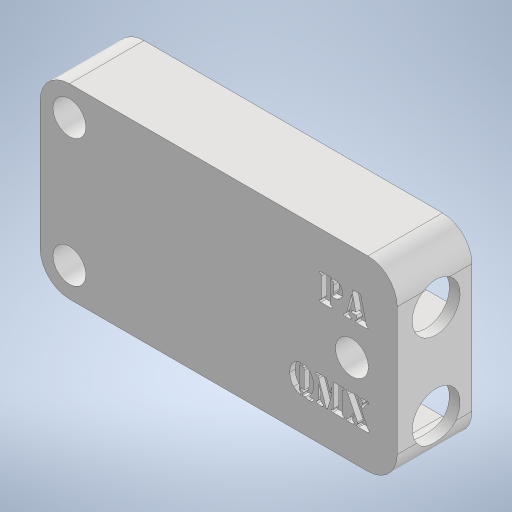
# Autodesk Inventor part: Case_Cap
Saved by Autodesk Inventor 2023 (Build 270158000, 158)
## iProperties
Created: 2024-10-24
Part Number: Case_Cap
Material: Generic
Document SubType Name: Modeling
Designer: lwerne
Density: 1 g/cm^3
Appearance: Default
Author: lwerne
Autodesk Inventor part; units mm, degrees
ref_plane "YZ Plane" through (0, 0, 0) normal (1, 0, 0) x (0, 1, 0)
ref_plane "XZ Plane" through (0, 0, 0) normal (0, 1, 0) x (-1, 0, 0)
ref_plane "XY Plane" through (0, 0, 0) normal (0, 0, 1) x (1, 0, 0)
sketch "Sketch1" plane through (0, 0, 0) normal (0, 0, 1) x (1, 0, 0)
  arc A0 (31.5, 12) -> (28, 15.5) centre (28, 12) ccw projected
  line L0 (31.5, 12) -> (31.5, -12) projected
  arc A1 (28, -15.5) -> (31.5, -12) centre (28, -12) ccw projected
  line L1 (28, -15.5) -> (-28, -15.5) projected
  arc A2 (-31.5, -12) -> (-28, -15.5) centre (-28, -12) ccw projected
  line L2 (-31.5, -12) -> (-31.5, 12) projected
  arc A3 (-28, 15.5) -> (-31.5, 12) centre (-28, 12) ccw projected
  line L3 (-28, 15.5) -> (28, 15.5) projected
  arc A4 (28, -17.5) -> (33.5, -12) centre (28, -12) ccw projected
  line L4 (33.5, 12) -> (33.5, -12) projected
  arc A5 (33.5, 12) -> (28, 17.5) centre (28, 12) ccw projected
  line L5 (-28, 17.5) -> (28, 17.5) projected
  arc A6 (-28, 17.5) -> (-33.5, 12) centre (-28, 12) ccw projected
  line L6 (-33.5, -12) -> (-33.5, 12) projected
  arc A7 (-33.5, -12) -> (-28, -17.5) centre (-28, -12) ccw projected
  line L7 (28, -17.5) -> (-28, -17.5) projected
  point P0 (0, 0)
extrude "Extrusion1" add sketch "Sketch1" along normal blind 12
ref_plane "Work Plane1" through (0, 0, 5.9) normal (0, 0, 1) x (1, 0, 0)
sketch "Sketch2" plane through (0, 0, 5.9) normal (0, 0, 1) x (1, 0, 0)
  circle A0 centre (-28, 12) radius 1.6 projected
  circle A1 centre (-28, -12) radius 1.6 projected
  circle A2 centre (25, -0.5) radius 1.6 projected
  line L0 (-28, 15.5) -> (28, 15.5) projected
  circle A3 centre (-28, 12) radius 3.5
  circle A4 centre (-28, -12) radius 3.5
  circle A5 centre (25, -0.5) radius 4
  line L1 (25, 3.5) -> (31.5, 3.5)
  line L2 (31.5, 12) -> (31.5, -12) projected
  line L3 (25, -4.5) -> (31.5, -4.5)
  line L4 (-28, -17.5) -> (28, -17.5) projected
  arc A6 (28, -17.5) -> (33.5, -12) centre (28, -12) ccw projected
  line L5 (33.5, -12) -> (33.5, 12) projected
  arc A7 (33.5, 12) -> (28, 17.5) centre (28, 12) ccw projected
  line L6 (28, 17.5) -> (-28, 17.5) projected
  arc A8 (-28, 17.5) -> (-33.5, 12) centre (-28, 12) ccw projected
  line L7 (-33.5, 12) -> (-33.5, -12) projected
  arc A9 (-33.5, -12) -> (-28, -17.5) centre (-28, -12) ccw projected
  line L8 (28, -15.5) -> (-28, -15.5) projected
  arc A10 (-31.5, -12) -> (-28, -15.5) centre (-28, -12) ccw projected
  line L9 (-31.5, -12) -> (-31.5, 12) projected
  arc A11 (-28, 15.5) -> (-31.5, 12) centre (-28, 12) ccw projected
  line L10 (-28, 15.5) -> (28, 15.5) projected
  arc A12 (31.5, 12) -> (28, 15.5) centre (28, 12) ccw projected
  line L11 (31.5, 12) -> (31.5, -12) projected
  arc A13 (28, -15.5) -> (31.5, -12) centre (28, -12) ccw projected
  circle A14 centre (-28, 12) radius 5.5
  circle A15 centre (-28, -12) radius 5.5
  point P0 (0, 0)
  point P1 (-23.7574, -15.5)
  point P2 (-31.5, -7.7574)
  point P3 (-31.5, 7.7574)
  point P4 (-23.7574, 15.5)
  point P5 (-31.5, 12)
  dimension "d2" = 8
  constraints: 4 centre point, 4 end point, 3 coincident, 2 point on circle, 2 point on line, 1 horizontal, 1 parallel, 3 other
  measures "d2" diameter of A5
ref_plane "Work Plane2" through (-31, -15, 0) normal (0, 0, 1) x (1, 0, 0)
extrude "Extrusion2" add sketch "Sketch2" against normal up to surface (5.9 mm away) contours L0 A14 L9 A3 | A3 | A15 L8 A4 L9 | L2 L3 A5 L1 | A4 | A5
sketch "Sketch3" plane through (0, 0, 5.9) normal (0, 0, 1) x (1, 0, 0)
  circle A0 centre (-28, 12) radius 1.6 projected
  circle A1 centre (-28, -12) radius 1.6 projected
  circle A2 centre (25, -0.5) radius 1.6 projected
  circle A3 centre (-28, 12) radius 3.1
  circle A4 centre (-28, -12) radius 1.6 projected
  circle A5 centre (-28, -12) radius 3.1
  circle A6 centre (25, -0.5) radius 1.6 projected
  circle A7 centre (25, -0.5) radius 3.1
  line L0 (31.5, 3.5) -> (31.5, -4.5) projected
  line L1 (31.5, 3.5) -> (25, 3.5) projected
  arc A8 (25, 3.5) -> (25, -4.5) centre (25, -0.5) ccw projected
  line L2 (25, -4.5) -> (31.5, -4.5) projected
  circle A9 centre (25, -0.5) radius 1.6 projected
  arc A10 (-31.5, -12) -> (-28, -15.5) centre (-28, -12) ccw projected
  circle A11 centre (-28, -12) radius 1.6 projected
  arc A12 (-28, 15.5) -> (-31.5, 12) centre (-28, 12) ccw projected
  circle A13 centre (-28, 12) radius 1.6 projected
  line L3 (-31.5, 7.7574) -> (-31.5, 12) projected
  arc A14 (-31.5, 7.7574) -> (-23.7574, 15.5) centre (-28, 12) ccw projected
  line L4 (-28, 15.5) -> (-23.7574, 15.5) projected
  line L5 (-23.7574, -15.5) -> (-28, -15.5) projected
  arc A15 (-23.7574, -15.5) -> (-31.5, -7.7574) centre (-28, -12) ccw projected
  line L6 (-31.5, -12) -> (-31.5, -7.7574) projected
  point P0 (0, 0)
  dimension "d5" = 6.2
  dimension "d6" = 6.2
  dimension "d7" = 6.2
  constraints: 3 centre point, 3 coincident
  measures "d5" diameter of A3
  measures "d6" diameter of A5
  measures "d7" diameter of A7
extrude "Extrusion3" add sketch "Sketch3" along normal up to surface (6.1 mm away) contours L0 L2 A8 L1 | L6 A15 L5 A10 | L4 A14 L3 A12
fillet "Fillet1" radius 2 4 edges at (-23.7574, -15.5, 6) (-31.5, -7.7574, 6) (-31.5, 7.7574, 6) (-23.7574, 15.5, 6)
sketch "Sketch4" plane through (0, 0, 12) normal (0, 0, 1) x (1, 0, 0)
  circle A0 centre (25, -0.5) radius 3.1 projected
  circle A1 centre (-28, 12) radius 3.1 projected
  circle A2 centre (-28, -12) radius 3.1 projected
  line L0 (-28, -17.5) -> (28, -17.5) projected
  arc A3 (28, -17.5) -> (33.5, -12) centre (28, -12) ccw projected
  line L1 (33.5, -12) -> (33.5, 12) projected
  arc A4 (33.5, 12) -> (28, 17.5) centre (28, 12) ccw projected
  line L2 (28, 17.5) -> (-28, 17.5) projected
  arc A5 (-28, 17.5) -> (-33.5, 12) centre (-28, 12) ccw projected
  line L3 (-33.5, 12) -> (-33.5, -12) projected
  arc A6 (-33.5, -12) -> (-28, -17.5) centre (-28, -12) ccw projected
  line L4 (-31.5, -4.6515) -> (-31.5, 4.6515) projected
  arc A7 (-29.1, 6.6111) -> (-31.5, 4.6515) centre (-29.5, 4.6515) ccw projected
  arc A8 (-29.1, 6.6111) -> (-22.6111, 13.1) centre (-28, 12) ccw projected
  arc A9 (-20.6515, 15.5) -> (-22.6111, 13.1) centre (-20.6515, 13.5) ccw projected
  line L5 (-20.6515, 15.5) -> (28, 15.5) construction
  arc A10 (31.5, 12) -> (28, 15.5) centre (28, 12) ccw projected
  line L6 (31.5, 12) -> (31.5, 3.5) projected
  line L7 (25, 3.5) -> (31.5, 3.5) projected
  arc A11 (25, 3.5) -> (25, -4.5) centre (25, -0.5) ccw projected
  line L8 (31.5, -4.5) -> (25, -4.5) projected
  line L9 (31.5, -4.5) -> (31.5, -12) projected
  arc A12 (28, -15.5) -> (31.5, -12) centre (28, -12) ccw projected
  line L10 (28, -15.5) -> (-20.6515, -15.5) projected
  arc A13 (-22.6111, -13.1) -> (-20.6515, -15.5) centre (-20.6515, -13.5) ccw projected
  arc A14 (-22.6111, -13.1) -> (-29.1, -6.6111) centre (-28, -12) ccw projected
  arc A15 (-31.5, -4.6515) -> (-29.1, -6.6111) centre (-29.5, -4.6515) ccw projected
  point P0 (0, 0)
sketch "Sketch5" plane through (0, 0, 12) normal (0, 0, 1) x (1, 0, 0)
  point P0 (0, 0)
extrude "Extrusion4" add sketch "Sketch4" along normal blind 2
sketch "Sketch6" plane through (33.5, -12, 0) normal (1, 0, 0) x (0, 0, -1)
  circle A0 centre (-6.7, 2.595) radius 3.2 projected
  circle A1 centre (-6.7, 20.267) radius 3.2 projected
  circle A2 centre (-6.7, 2.595) radius 4.5
  circle A3 centre (-6.7, 20.267) radius 4.5
  point P0 (0, 12)
  dimension "d13" = 9
  dimension "d14" = 9
  constraints: 2 centre point, 2 coincident
  measures "d13" diameter of A2
  measures "d14" diameter of A3
extrude "Extrusion5" cut sketch "Sketch6" against normal blind 5.9375 contours A0 | A1 | A2 | A3
sketch "Sketch7" plane through (-33.5, -12, 0) normal (-1, 0, 0) x (0, 0, 1)
  arc A0 (1.2, 17.6122) -> (0.07, 16.4822) centre (1.2, 16.4822) ccw projected
  arc A1 (0.07, 10.0022) -> (1.2, 8.8722) centre (1.2, 10.0022) ccw projected
  arc A2 (1.9, 8.8722) -> (3.03, 10.0022) centre (1.9, 10.0022) ccw projected
  line L0 (0, 13.1) -> (5.9, 13.1) projected
  line L1 (0, 24) -> (0, 0) projected
  line L2 (0, 7.3485) -> (0, 16.6515) projected
  line L3 (0, 17.6122) -> (0, 8.8722)
  line L4 (0, 8.8722) -> (3.03, 8.8722)
  line L5 (3.03, 8.8722) -> (3.03, 17.6122)
  line L6 (3.03, 17.6122) -> (0, 17.6122)
  line L7 (-2.485, 20.7422) -> (5.515, 20.7422)
  line L8 (5.515, 20.7422) -> (5.515, 5.7422)
  line L9 (5.515, 5.7422) -> (-2.485, 5.7422)
  line L10 (-2.485, 5.7422) -> (-2.485, 20.7422)
  line L11 (-2.485, 20.7422) -> (5.515, 5.7422) construction
  line L12 (5.515, 20.7422) -> (-2.485, 5.7422) construction
  point P0 (1.515, 13.2422)
  point P1 (0, 5.7422)
  point P2 (0, 20.7422)
  dimension "d17" = 8
  dimension "d18" = 15
  constraints: 20 end point, 4 parallel, 2 midpoint, 2 perpendicular, 2 point on line, 1 horizontal
  measures "d17" distance of L8.end L9.end
  measures "d18" distance of L7.end L8.end
extrude "Extrusion6" cut sketch "Sketch7" against normal blind 11.525 contours L4 L1 L0 L5 A2 | L4 L5 L0 L8 L9 L1 | A2 L5 L4 | L5 L6 L1 L7 L8 L0 | L0 L1 L6 L5
fillet "Fillet2" radius 2 2 edges at (-28.5343, 8.7422, 5.515) (-32.0958, -6.2578, 5.515)
sketch "Sketch8" plane through (0, 0, 14) normal (0, 0, 1) x (1, 0, 0)
  line L0 (13.173, -6.1079) -> (28.4117, -6.1079) construction
  line L1 (28.4117, -6.1079) -> (28.4117, -11.4638) construction
  line L2 (28.4117, -11.4638) -> (13.173, -11.4638) construction
  line L3 (13.173, -11.4638) -> (13.173, -6.1079) construction
  line L4 (18.6124, 10.5749) -> (28.0308, 10.5749) construction
  line L5 (28.0308, 10.5749) -> (28.0308, 5.5749) construction
  line L6 (28.0308, 5.5749) -> (18.6124, 5.5749) construction
  line L7 (18.6124, 5.5749) -> (18.6124, 10.5749) construction
  line L8 (20.9127, 10.5749) -> (20.9127, 6.2693)
  spline S0 degree 2 poles (20.9127, 6.2693) (20.9127, 6.1261) (20.9692, 6.0653) knots 0 0 0 1 1 1
  spline S1 degree 2 poles (20.9692, 6.0653) (20.9952, 6.0306) (21.0473, 6.0089) (21.1905, 5.9742) knots 0 0 0 1 2 2 2
  spline S2 degree 2 poles (21.1905, 5.9742) (21.3685, 5.9351) (21.3685, 5.7745) knots 0 0 0 1 1 1
  spline S3 degree 2 poles (21.3685, 5.7745) (21.3685, 5.679) (21.273, 5.6183) knots 0 0 0 1 1 1
  spline S4 degree 2 poles (21.273, 5.6183) (21.2035, 5.5749) (21.0429, 5.5749) knots 0 0 0 1 1 1
  line L9 (21.0429, 5.5749) -> (20.9171, 5.5749)
  line L10 (20.9171, 5.5749) -> (19.2808, 5.5749)
  line L11 (19.2808, 5.5749) -> (19.1853, 5.5749)
  spline S5 degree 2 poles (19.1853, 5.5749) (19.0551, 5.5749) (18.9119, 5.6747) (18.9119, 5.7658) knots 0 0 0 1 2 2 2
  spline S6 degree 2 poles (18.9119, 5.7658) (18.9119, 5.9134) (19.0594, 5.9612) knots 0 0 0 1 1 1
  spline S7 degree 2 poles (19.0594, 5.9612) (19.181, 6.0046) (19.22, 6.0219) (19.2417, 6.0566) knots 0 0 0 1 2 2 2
  spline S8 degree 2 poles (19.2417, 6.0566) (19.2851, 6.1131) (19.2851, 6.2433) knots 0 0 0 1 1 1
  line L12 (19.2851, 6.2433) -> (19.2851, 9.9065)
  spline S9 degree 2 poles (19.2851, 9.9065) (19.2851, 10.0367) (19.2417, 10.0931) knots 0 0 0 1 1 1
  spline S10 degree 2 poles (19.2417, 10.0931) (19.22, 10.1278) (19.181, 10.1452) (19.0594, 10.1842) knots 0 0 0 1 2 2 2
  spline S11 degree 2 poles (19.0594, 10.1842) (18.9119, 10.232) (18.9119, 10.3839) knots 0 0 0 1 1 1
  spline S12 degree 2 poles (18.9119, 10.3839) (18.9119, 10.475) (19.0551, 10.5749) (19.1853, 10.5749) knots 0 0 0 1 2 2 2
  line L13 (19.1853, 10.5749) -> (19.2808, 10.5749)
  line L14 (19.2808, 10.5749) -> (20.9127, 10.5749)
  line L15 (21.2252, 7.4889) -> (21.2252, 7.8796)
  spline S13 degree 2 poles (21.2252, 7.8796) (21.3815, 7.9186) (21.5073, 7.9967) (21.5551, 8.0836) knots 0 0 0 1 2 2 2
  spline S14 degree 2 poles (21.5551, 8.0836) (21.6332, 8.2268) (21.6332, 8.4655) knots 0 0 0 1 1 1
  line L16 (21.6332, 8.4655) -> (21.6332, 9.6417)
  spline S15 degree 2 poles (21.6332, 9.6417) (21.6332, 9.8153) (21.5811, 9.9803) (21.503, 10.0497) knots 0 0 0 1 2 2 2
  spline S16 degree 2 poles (21.503, 10.0497) (21.3988, 10.1539) (21.2209, 10.1799) knots 0 0 0 1 1 1
  line L17 (21.2209, 10.1799) -> (21.2209, 10.5749)
  spline S17 degree 2 poles (21.2209, 10.5749) (21.9761, 10.5749) (22.332, 10.4316) knots 0 0 0 1 1 1
  spline S18 degree 2 poles (22.332, 10.4316) (22.7487, 10.2667) (22.9874, 9.9282) knots 0 0 0 1 1 1
  spline S19 degree 2 poles (22.9874, 9.9282) (23.2348, 9.5766) (23.2348, 9.0731) knots 0 0 0 1 1 1
  spline S20 degree 2 poles (23.2348, 9.0731) (23.2348, 8.5089) (22.9874, 8.1487) knots 0 0 0 1 1 1
  spline S21 degree 2 poles (22.9874, 8.1487) (22.7356, 7.7928) (22.2886, 7.6235) knots 0 0 0 1 1 1
  spline S22 degree 2 poles (22.2886, 7.6235) (21.9197, 7.4889) (21.2252, 7.4889) knots 0 0 0 1 1 1
  line L18 (25.1575, 10.5749) -> (26.6332, 10.5749)
  line L19 (26.6332, 10.5749) -> (27.6488, 6.2693)
  spline S23 degree 2 poles (27.6488, 6.2693) (27.6792, 6.1565) (27.7139, 6.0697) knots 0 0 0 1 1 1
  spline S24 degree 2 poles (27.7139, 6.0697) (27.7487, 6.0002) (27.8615, 5.9568) knots 0 0 0 1 1 1
  spline S25 degree 2 poles (27.8615, 5.9568) (27.957, 5.9134) (28.0308, 5.8353) (28.0308, 5.7658) knots 0 0 0 1 2 2 2
  spline S26 degree 2 poles (28.0308, 5.7658) (28.0308, 5.5749) (27.7443, 5.5749) knots 0 0 0 1 1 1
  line L20 (27.7443, 5.5749) -> (25.9171, 5.5749)
  spline S27 degree 2 poles (25.9171, 5.5749) (25.8086, 5.5749) (25.674, 5.6834) (25.674, 5.7702) knots 0 0 0 1 2 2 2
  spline S28 degree 2 poles (25.674, 5.7702) (25.674, 5.844) (25.7348, 5.9178) (25.8346, 5.9698) knots 0 0 0 1 2 2 2
  spline S29 degree 2 poles (25.8346, 5.9698) (25.9084, 6.0089) (25.9692, 6.0957) (25.9692, 6.1608) knots 0 0 0 1 2 2 2
  spline S30 degree 2 poles (25.9692, 6.1608) (25.9692, 6.2259) (25.9561, 6.2737) knots 0 0 0 1 1 1
  line L21 (25.9561, 6.2737) -> (25.8389, 6.8032)
  line L22 (25.8389, 6.8032) -> (24.819, 6.8032)
  line L23 (24.819, 6.8032) -> (24.9188, 7.2372)
  line L24 (24.9188, 7.2372) -> (25.7391, 7.2372)
  line L25 (25.7391, 7.2372) -> (25.062, 10.2146)
  line L26 (25.062, 10.2146) -> (25.1575, 10.5749)
  line L27 (24.9014, 9.6417) -> (25.0881, 8.8865)
  line L28 (25.0881, 8.8865) -> (24.4414, 6.5211)
  spline S31 degree 2 poles (24.4414, 6.5211) (24.411, 6.4169) (24.411, 6.3301) knots 0 0 0 1 1 1
  spline S32 degree 2 poles (24.411, 6.3301) (24.411, 6.1) (24.628, 6.0002) knots 0 0 0 1 1 1
  line L29 (24.628, 6.0002) -> (24.7539, 5.9395)
  spline S33 degree 2 poles (24.7539, 5.9395) (24.8754, 5.8874) (24.8754, 5.7572) knots 0 0 0 1 1 1
  spline S34 degree 2 poles (24.8754, 5.7572) (24.8754, 5.5749) (24.6106, 5.5749) knots 0 0 0 1 1 1
  line L30 (24.6106, 5.5749) -> (23.6818, 5.5749)
  spline S35 degree 2 poles (23.6818, 5.5749) (23.5429, 5.5749) (23.3867, 5.6877) (23.3867, 5.7875) knots 0 0 0 1 2 2 2
  spline S36 degree 2 poles (23.3867, 5.7875) (23.3867, 5.8917) (23.5473, 5.9612) knots 0 0 0 1 1 1
  spline S37 degree 2 poles (23.5473, 5.9612) (23.6992, 6.0306) (23.8424, 6.1348) (23.9075, 6.2259) knots 0 0 0 1 2 2 2
  spline S38 degree 2 poles (23.9075, 6.2259) (24.0073, 6.3778) (24.0768, 6.6252) knots 0 0 0 1 1 1
  line L31 (24.0768, 6.6252) -> (24.9014, 9.6417)
  spline S39 degree 2 poles (16.9881, -10.7911) (17.1227, -10.9256) (17.344, -10.9256) knots 0 0 0 1 1 1
  spline S40 degree 2 poles (17.344, -10.9256) (17.4742, -10.9256) (17.5784, -10.8779) knots 0 0 0 1 1 1
  spline S41 degree 2 poles (17.5784, -10.8779) (17.6695, -10.8388) (17.7043, -10.8388) knots 0 0 0 1 1 1
  spline S42 degree 2 poles (17.7043, -10.8388) (17.7477, -10.8388) (17.8258, -10.9386) (17.8258, -10.9951) knots 0 0 0 1 2 2 2
  spline S43 degree 2 poles (17.8258, -10.9951) (17.8258, -11.1122) (17.6522, -11.2424) knots 0 0 0 1 1 1
  spline S44 degree 2 poles (17.6522, -11.2424) (17.3353, -11.4638) (17.0011, -11.4638) knots 0 0 0 1 1 1
  spline S45 degree 2 poles (17.0011, -11.4638) (16.5628, -11.4638) (16.3023, -11.1947) knots 0 0 0 1 1 1
  spline S46 degree 2 poles (16.3023, -11.1947) (16.055, -11.2815) (15.7208, -11.3119) knots 0 0 0 1 1 1
  line L32 (15.7208, -11.3119) -> (15.7208, -10.9039)
  spline S47 degree 2 poles (15.7208, -10.9039) (15.8032, -10.8865) (15.8813, -10.8431) (15.9291, -10.7997) knots 0 0 0 1 2 2 2
  line L33 (15.9291, -10.7997) -> (15.8987, -10.7694)
  spline S48 degree 2 poles (15.8987, -10.7694) (15.7989, -10.6478) (15.673, -10.5567) (15.5862, -10.5437) knots 0 0 0 1 2 2 2
  spline S49 degree 2 poles (15.5862, -10.5437) (15.4734, -10.5176) (15.4126, -10.4959) (15.3865, -10.4612) knots 0 0 0 1 2 2 2
  spline S50 degree 2 poles (15.3865, -10.4612) (15.3518, -10.4178) (15.3518, -10.357) knots 0 0 0 1 1 1
  spline S51 degree 2 poles (15.3518, -10.357) (15.3518, -10.2529) (15.5298, -10.1357) (15.6773, -10.1357) knots 0 0 0 1 2 2 2
  spline S52 degree 2 poles (15.6773, -10.1357) (15.7989, -10.1357) (15.9725, -10.1791) (16.068, -10.2355) knots 0 0 0 1 2 2 2
  line L34 (16.068, -10.2355) -> (16.068, -7.0194)
  spline S53 degree 2 poles (16.068, -7.0194) (16.068, -6.824) (16.0029, -6.7112) knots 0 0 0 1 1 1
  spline S54 degree 2 poles (16.0029, -6.7112) (15.9551, -6.6331) (15.8336, -6.5463) (15.7208, -6.5029) knots 0 0 0 1 2 2 2
  line L35 (15.7208, -6.5029) -> (15.7208, -6.1079)
  spline S55 degree 2 poles (15.7208, -6.1079) (16.1157, -6.1253) (16.7754, -6.4117) (17.0576, -6.6895) knots 0 0 0 1 2 2 2
  spline S56 degree 2 poles (17.0576, -6.6895) (17.8041, -7.4187) (17.8041, -8.7164) knots 0 0 0 1 1 1
  spline S57 degree 2 poles (17.8041, -8.7164) (17.8041, -10.0532) (16.9881, -10.7911) knots 0 0 0 1 1 1
  spline S58 degree 2 poles (15.4213, -6.5029) (15.2346, -6.5723) (15.0827, -6.798) (15.0827, -7.0194) knots 0 0 0 1 2 2 2
  line L36 (15.0827, -7.0194) -> (15.0827, -10.2919)
  spline S59 degree 2 poles (15.0827, -10.2919) (15.0827, -10.6131) (15.1695, -10.7477) knots 0 0 0 1 1 1
  spline S60 degree 2 poles (15.1695, -10.7477) (15.239, -10.8562) (15.4213, -10.9039) knots 0 0 0 1 1 1
  line L37 (15.4213, -10.9039) -> (15.4213, -11.3076)
  spline S61 degree 2 poles (15.4213, -11.3076) (14.6096, -11.2424) (14.0584, -10.6956) knots 0 0 0 1 1 1
  spline S62 degree 2 poles (14.0584, -10.6956) (13.3466, -9.9838) (13.3466, -8.7121) knots 0 0 0 1 1 1
  spline S63 degree 2 poles (13.3466, -8.7121) (13.3466, -8.074) (13.7242, -7.0454) (14.0931, -6.6895) knots 0 0 0 1 2 2 2
  spline S64 degree 2 poles (14.0931, -6.6895) (14.3753, -6.4117) (15.0263, -6.1253) (15.4213, -6.1079) knots 0 0 0 1 2 2 2
  line L38 (15.4213, -6.1079) -> (15.4213, -6.5029)
  line L39 (21.5454, -6.2077) -> (23.173, -6.2077)
  line L40 (23.173, -6.2077) -> (23.2728, -6.2077)
  spline S65 degree 2 poles (23.2728, -6.2077) (23.5463, -6.2077) (23.5463, -6.3987) knots 0 0 0 1 1 1
  spline S66 degree 2 poles (23.5463, -6.3987) (23.5463, -6.5506) (23.3987, -6.5984) knots 0 0 0 1 1 1
  spline S67 degree 2 poles (23.3987, -6.5984) (23.2772, -6.6374) (23.2381, -6.6548) (23.2164, -6.6895) knots 0 0 0 1 2 2 2
  spline S68 degree 2 poles (23.2164, -6.6895) (23.173, -6.7459) (23.173, -6.8761) knots 0 0 0 1 1 1
  line L41 (23.173, -6.8761) -> (23.173, -10.5393)
  spline S69 degree 2 poles (23.173, -10.5393) (23.173, -10.6695) (23.2164, -10.726) knots 0 0 0 1 1 1
  spline S70 degree 2 poles (23.2164, -10.726) (23.2381, -10.7607) (23.2772, -10.778) (23.3987, -10.8214) knots 0 0 0 1 2 2 2
  spline S71 degree 2 poles (23.3987, -10.8214) (23.5463, -10.8692) (23.5463, -11.0168) knots 0 0 0 1 1 1
  spline S72 degree 2 poles (23.5463, -11.0168) (23.5463, -11.2077) (23.2728, -11.2077) knots 0 0 0 1 1 1
  line L42 (23.2728, -11.2077) -> (23.173, -11.2077)
  line L43 (23.173, -11.2077) -> (21.5411, -11.2077)
  line L44 (21.5411, -11.2077) -> (21.4195, -11.2077)
  spline S73 degree 2 poles (21.4195, -11.2077) (21.2589, -11.2077) (21.094, -11.1079) (21.094, -11.0081) knots 0 0 0 1 2 2 2
  spline S74 degree 2 poles (21.094, -11.0081) (21.094, -10.8475) (21.272, -10.8084) knots 0 0 0 1 1 1
  spline S75 degree 2 poles (21.272, -10.8084) (21.4152, -10.7737) (21.4629, -10.752) (21.489, -10.7216) knots 0 0 0 1 2 2 2
  spline S76 degree 2 poles (21.489, -10.7216) (21.5454, -10.6565) (21.5454, -10.5133) knots 0 0 0 1 1 1
  line L45 (21.5454, -10.5133) -> (21.5454, -6.2077)
  line L46 (20.1999, -6.2077) -> (20.9247, -8.265)
  line L47 (20.9247, -8.265) -> (21.2416, -7.1539)
  line L48 (21.2416, -7.1539) -> (21.2416, -8.3692)
  line L49 (21.2416, -8.3692) -> (20.3952, -11.2077)
  line L50 (20.3952, -11.2077) -> (20.1999, -11.2077)
  line L51 (20.1999, -11.2077) -> (18.7806, -6.9933)
  spline S77 degree 2 poles (18.7806, -6.9933) (18.7069, -6.7806) (18.6287, -6.7069) knots 0 0 0 1 1 1
  spline S78 degree 2 poles (18.6287, -6.7069) (18.581, -6.6591) (18.4638, -6.6374) knots 0 0 0 1 1 1
  spline S79 degree 2 poles (18.4638, -6.6374) (18.2251, -6.5853) (18.2251, -6.4074) knots 0 0 0 1 1 1
  spline S80 degree 2 poles (18.2251, -6.4074) (18.2251, -6.3119) (18.3596, -6.2077) (18.4898, -6.2077) knots 0 0 0 1 2 2 2
  line L52 (18.4898, -6.2077) -> (20.1999, -6.2077)
  line L53 (18.7806, -7.8961) -> (19.1669, -8.9985)
  line L54 (19.1669, -8.9985) -> (19.1669, -10.101)
  spline S81 degree 2 poles (19.1669, -10.101) (19.1669, -10.2702) (19.193, -10.4178) (19.2364, -10.5046) knots 0 0 0 1 2 2 2
  spline S82 degree 2 poles (19.2364, -10.5046) (19.3145, -10.6652) (19.449, -10.7477) knots 0 0 0 1 1 1
  line L55 (19.449, -10.7477) -> (19.5836, -10.8345)
  spline S83 degree 2 poles (19.5836, -10.8345) (19.7225, -10.9169) (19.7225, -11.0211) knots 0 0 0 1 1 1
  spline S84 degree 2 poles (19.7225, -11.0211) (19.7225, -11.2077) (19.449, -11.2077) knots 0 0 0 1 1 1
  line L56 (19.449, -11.2077) -> (18.5333, -11.2077)
  spline S85 degree 2 poles (18.5333, -11.2077) (18.2555, -11.2077) (18.2555, -11.0254) knots 0 0 0 1 1 1
  spline S86 degree 2 poles (18.2555, -11.0254) (18.2555, -10.9647) (18.3032, -10.9039) (18.3727, -10.8648) knots 0 0 0 1 2 2 2
  spline S87 degree 2 poles (18.3727, -10.8648) (18.7806, -10.6435) (18.7806, -10.101) knots 0 0 0 1 1 1
  line L57 (18.7806, -10.101) -> (18.7806, -7.8961)
  line L58 (26.1461, -6.8501) -> (27.9907, -10.5957)
  spline S88 degree 2 poles (27.9907, -10.5957) (28.0558, -10.726) (28.1687, -10.7824) knots 0 0 0 1 1 1
  spline S89 degree 2 poles (28.1687, -10.7824) (28.2685, -10.8345) (28.3379, -10.9213) (28.3379, -10.9994) knots 0 0 0 1 2 2 2
  spline S90 degree 2 poles (28.3379, -10.9994) (28.3379, -11.0992) (28.2642, -11.1556) knots 0 0 0 1 1 1
  spline S91 degree 2 poles (28.2642, -11.1556) (28.2034, -11.2077) (27.9994, -11.2077) knots 0 0 0 1 1 1
  line L59 (27.9994, -11.2077) -> (26.2806, -11.2077)
  spline S92 degree 2 poles (26.2806, -11.2077) (26.0853, -11.2077) (26.0246, -11.1817) knots 0 0 0 1 1 1
  spline S93 degree 2 poles (26.0246, -11.1817) (25.8987, -11.1253) (25.8987, -10.9951) knots 0 0 0 1 1 1
  spline S94 degree 2 poles (25.8987, -10.9951) (25.8987, -10.9473) (25.9508, -10.8779) (26.0202, -10.8258) knots 0 0 0 1 2 2 2
  spline S95 degree 2 poles (26.0202, -10.8258) (26.1418, -10.7346) (26.1374, -10.6565) knots 0 0 0 1 1 1
  spline S96 degree 2 poles (26.1374, -10.6565) (26.1331, -10.5957) (26.0723, -10.4699) knots 0 0 0 1 1 1
  line L60 (26.0723, -10.4699) -> (24.2754, -6.8501)
  spline S97 degree 2 poles (24.2754, -6.8501) (24.232, -6.7589) (24.1279, -6.6504) (24.0454, -6.607) knots 0 0 0 1 2 2 2
  spline S98 degree 2 poles (24.0454, -6.607) (23.9716, -6.5723) (23.9152, -6.4812) (23.9152, -6.4074) knots 0 0 0 1 2 2 2
  spline S99 degree 2 poles (23.9152, -6.4074) (23.9152, -6.2945) (24.0714, -6.2077) (24.2754, -6.2077) knots 0 0 0 1 2 2 2
  line L61 (24.2754, -6.2077) -> (25.9812, -6.2077)
  spline S100 degree 2 poles (25.9812, -6.2077) (26.1678, -6.2077) (26.3327, -6.3032) (26.3327, -6.4074) knots 0 0 0 1 2 2 2
  spline S101 degree 2 poles (26.3327, -6.4074) (26.3327, -6.5159) (26.2112, -6.594) knots 0 0 0 1 1 1
  spline S102 degree 2 poles (26.2112, -6.594) (26.1548, -6.6374) (26.1157, -6.6895) (26.1157, -6.7372) knots 0 0 0 1 2 2 2
  spline S103 degree 2 poles (26.1157, -6.7372) (26.1157, -6.7893) (26.1461, -6.8501) knots 0 0 0 1 1 1
  line L62 (25.2433, -9.4195) -> (25.443, -9.8362)
  line L63 (25.443, -9.8362) -> (25.2173, -10.2095)
  spline S104 degree 2 poles (25.2173, -10.2095) (25.0914, -10.4135) (25.0914, -10.535) knots 0 0 0 1 1 1
  spline S105 degree 2 poles (25.0914, -10.535) (25.0914, -10.7086) (25.2867, -10.7911) knots 0 0 0 1 1 1
  spline S106 degree 2 poles (25.2867, -10.7911) (25.3996, -10.8345) (25.4777, -10.9213) (25.4777, -10.9994) knots 0 0 0 1 2 2 2
  spline S107 degree 2 poles (25.4777, -10.9994) (25.4777, -11.1036) (25.3909, -11.1687) knots 0 0 0 1 1 1
  spline S108 degree 2 poles (25.3909, -11.1687) (25.3562, -11.1947) (25.278, -11.2077) (25.1652, -11.2077) knots 0 0 0 1 2 2 2
  line L64 (25.1652, -11.2077) -> (24.219, -11.2077)
  spline S109 degree 2 poles (24.219, -11.2077) (24.1018, -11.2077) (23.9673, -11.1079) (23.9673, -11.0211) knots 0 0 0 1 2 2 2
  spline S110 degree 2 poles (23.9673, -11.0211) (23.9673, -10.9516) (24.0497, -10.8605) (24.1583, -10.8214) knots 0 0 0 1 2 2 2
  spline S111 degree 2 poles (24.1583, -10.8214) (24.4317, -10.7129) (24.5836, -10.4699) knots 0 0 0 1 1 1
  line L65 (24.5836, -10.4699) -> (25.2433, -9.4195)
  line L66 (26.9708, -7.8657) -> (26.7668, -7.4577)
  line L67 (26.7668, -7.4577) -> (26.9708, -7.1105)
  spline S112 degree 2 poles (26.9708, -7.1105) (27.0402, -6.989) (27.0402, -6.9022) knots 0 0 0 1 1 1
  spline S113 degree 2 poles (27.0402, -6.9022) (27.0402, -6.8197) (26.9404, -6.6678) (26.8622, -6.6287) knots 0 0 0 1 2 2 2
  line L68 (26.8622, -6.6287) -> (26.732, -6.5723)
  spline S114 degree 2 poles (26.732, -6.5723) (26.6973, -6.5506) (26.6409, -6.4508) (26.6409, -6.3987) knots 0 0 0 1 2 2 2
  spline S115 degree 2 poles (26.6409, -6.3987) (26.6409, -6.3119) (26.7668, -6.2077) (26.8666, -6.2077) knots 0 0 0 1 2 2 2
  line L69 (26.8666, -6.2077) -> (27.9256, -6.2077)
  spline S116 degree 2 poles (27.9256, -6.2077) (28.0298, -6.2077) (28.1643, -6.2989) (28.1643, -6.3727) knots 0 0 0 1 2 2 2
  spline S117 degree 2 poles (28.1643, -6.3727) (28.1643, -6.4595) (28.0992, -6.5246) knots 0 0 0 1 1 1
  spline S118 degree 2 poles (28.0992, -6.5246) (28.0732, -6.5506) (27.943, -6.6201) knots 0 0 0 1 1 1
  spline S119 degree 2 poles (27.943, -6.6201) (27.6826, -6.7633) (27.5133, -7.0324) knots 0 0 0 1 1 1
  line L70 (27.5133, -7.0324) -> (26.9708, -7.8657)
  point P0 (0, 0)
  constraints: 4 other
extrude "Extrusion7" cut sketch "Sketch8" against normal blind 1
body "Solid1"
